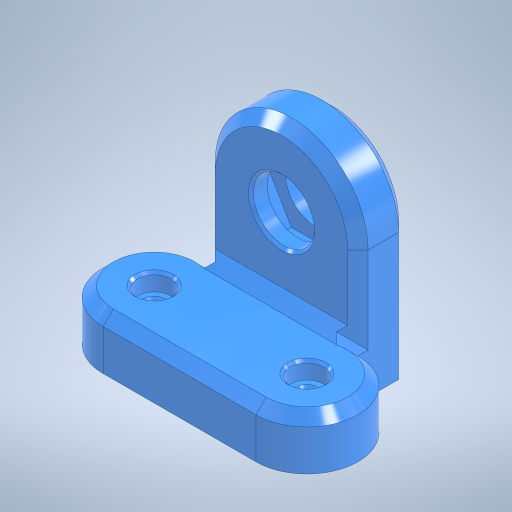
# Autodesk Inventor part: Sensorhalter_Portal
Saved by Autodesk Inventor 2024 (Build 280153020, 153B)
## iProperties
Created: 2023-08-03
Part Number: Sensorhalter_Portal
Material: PC/ABS-Kunststoff
Document SubType Name: Modeling
Designer: hol
Density: 1.1 g/cm^3
Appearance: Cyan
Author: hol
Autodesk Inventor part; units mm, degrees
ref_plane "YZ Plane" through (0, 0, 0) normal (1, 0, 0) x (0, 1, 0)
ref_plane "XZ Plane" through (0, 0, 0) normal (0, 1, 0) x (-1, 0, 0)
sketch "Skizze1" plane through (0, 0, 0) normal (1, 0, 0) x (0, 1, 0)
  line L0 (0, 0) -> (0, -30)
  line L1 (0, -30) -> (40, -30)
  line L2 (40, -30) -> (40, -20)
  line L3 (40, -20) -> (10, -20)
  line L4 (10, -20) -> (10, 0)
  line L5 (10, 0) -> (0, 0)
  dimension "d0" = 40
  dimension "d1" = 30
  dimension "d2" = 10
  dimension "d3" = 10
  constraints: 12 end point, 5 perpendicular, 1 vertical
  measures "d0" distance of L0.end L1.end
  measures "d1" distance of L0.start L0.end
  measures "d2" distance of L1.end L2.end
  measures "d3" distance of L4.end L0.start
extrude "Extrusion1" add sketch "Skizze1" along normal blind 30
ref_plane "Arbeitsebene1" through (0, 10, -25) normal (0, 0, 1) x (1, 0, 0)
sketch "Skizze2" plane through (0, 10, -25) normal (0, 0, 1) x (1, 0, 0)
  line L0 (0, -10) -> (0, 30) projected
  line L1 (0, 30) -> (30, 30) projected
  line L2 (30, -10) -> (30, 30) projected
  line L3 (0, 30) -> (30, 0) construction
  line L4 (30, 30) -> (0, 0) construction
  line L5 (0, 0) -> (30, 0) construction
  line L6 (5.2428, 15) -> (10.1214, 23.45)
  line L7 (10.1214, 23.45) -> (19.8786, 23.45)
  line L8 (19.8786, 23.45) -> (24.7572, 15)
  line L9 (24.7572, 15) -> (19.8786, 6.55)
  line L10 (19.8786, 6.55) -> (10.1214, 6.55)
  line L11 (10.1214, 6.55) -> (5.2428, 15)
  circle A0 centre (15, 15) radius 6
  dimension "d6" = 16.9
  dimension "d9" = 12
  constraints: 16 end point, 1 centre point, 1 coincident, 1 midpoint, 13 other
  measures "d6" distance between parallel lines of L9 L6
  measures "d9" diameter of A0
extrude "Extrusion2" cut sketch "Skizze2" along normal mid plane 3.6
extrude "Extrusion3" cut sketch "Skizze2" along normal mid plane 10 contours A0
sketch "Skizze3" plane through (0, 10, 0) normal (0, 1, 0) x (1, 0, 0)
  line L0 (0, 20) -> (0, 0) projected
  line L1 (0, 0) -> (30, 0) projected
  line L2 (30, 20) -> (30, 0) projected
  line L3 (0, 20) -> (30, 20) projected
  arc A0 (0, 20) -> (0, 0) centre (0, 10) ccw
  arc A1 (30, 0) -> (30, 20) centre (30, 10) ccw
  point P0 (0, 0)
  constraints: 4 point on circle, 4 tangent, 2 centre point
extrude "Extrusion4" add sketch "Skizze3" against normal up to surface (10 mm away) contours L0 A0 | A1 L2
hole "Bohrung1" at (0, 10, -10) at (30, 10, -10) direction (0, -1, 0) diameter 3.4 end through all counterbore diameter 6.5 counterbore depth 3.4 clearance for "Inbusschraube ISO 4762" size "M3" standard "ISO"
fillet "Rundung1" radius 15 2 edges at (30, 40, -25) (0, 40, -25)
chamfer "Fasen1" distance 2 angle 45 9 edges at (15, 10, 0) (40, 10, -10) (-10, 10, -10) (30, 17.5001, -20) (25.6066, 35.6066, -20) (0, 17.5001, -20) (30, 12.5001, -30) (25.6066, 35.6066, -30) (0, 12.5001, -30)
chamfer "Fasen2" distance 2 angle 45 2 edges at (30, 10, -20) (0, 10, -20)
chamfer "Fasen3" distance 0.5 angle 45 6 edges at (0, 10, -13.25) (30, 10, -13.25) (0, 6.6, -11.7) (30, 6.6, -11.7) (9, 25, -20) (9, 25, -30)
chamfer "Fasen4" distance 2.2 angle 45 1 edges at (15, 10, -20)
